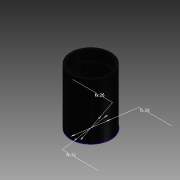
# Autodesk Inventor part: CsapágyHáz
Saved by Autodesk Inventor 2015 (Build 190159000, 159)
## iProperties
Created: 2014-08-08
Part Number: CsapágyHáz
Material: Acetal Resin, Black
Document SubType Name: Modeling
Designer: laca
Density: 1.425 g/cm^3
Appearance: Smooth - Black
Mass: 15.5926 g
Surface Area: 88.4672 cm^2
Volume: 10.9422 cm^3
Author: laca
Autodesk Inventor part; units mm, degrees
ref_plane "YZ Plane" through (0, 0, 0) normal (1, 0, 0) x (0, 1, 0)
ref_plane "XZ Plane" through (0, 0, 0) normal (0, 1, 0) x (-1, 0, 0)
ref_plane "XY Plane" through (0, 0, 0) normal (0, 0, 1) x (1, 0, 0)
sketch "Sketch1" plane through (0, 0, 0) normal (0, 1, 0) x (-1, 0, 0)
  circle A0 centre (0, 0) radius 14
  circle A1 centre (0, 0) radius 13
  circle A2 centre (0, 0) radius 16
  dimension "d0" = 26
  dimension "d1" = 28
  dimension "d2" = 32
  constraints: 3 centre point, 3 coincident
  measures "d0" diameter of A1
  measures "d1" diameter of A0
  measures "d2" diameter of A2
extrude "Extrusion1" add sketch "Sketch1" along normal blind 22.5 contours A0 | A2
extrude "Extrusion2" cut sketch "Sketch1" along normal blind 8 contours A0
mirror "Mirror1" about plane through (0, 22.5, 0) normal (0, 1, 0)
equation "\"d0\" = CsapágyHázBelsőÁtmérő"
equation "\"d1\" = CsapágyKülsőÁtmérő"
equation "\"d2\" = CsapágyHázKülsőÁtmérő"
equation "\"d3\" = 0.5 * CsapágyHázHoszza"
equation "\"d5\" = CsapágySzélesége"
equation "\"ZártSzelvényFalVastagság\" = 1.5"
equation "\"ZártSzelvényBelsőÁtmérő\" = 12"
equation "\"ZártSzelvényKülsőÁtmérő\" = 15"
equation "\"CsapágyBelsőÁtmérő\" = 12"
equation "\"CsapágySzélesége\" = 8"
equation "\"CsapágyKülsőÁtmérő\" = 28"
equation "\"CsapágyHázBelsőÁtmérő\" = 26"
equation "\"CsapágyHázHoszza\" = 45"
equation "\"CsapágyHázKülsőÁtmérő\" = 32"
body "Solid1"
